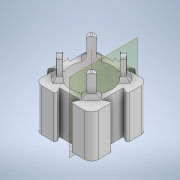
# Autodesk Inventor part: 4x11mmFlatBottom
Saved by Autodesk Inventor 2022.2 (Build 262287010, 287A)
## iProperties
Part Number: 4x11mmFlatBottom
Material: Generic
Document SubType Name: Modeling
Designer: yiunf
Appearance: Default
Author: yiunf
## iProperties of the stored document 4x11mm_3DPrint.ipt
Part Number: 4x11mm_3DPrint
Material: Generic
Document SubType Name: Modeling
Designer: yiunf
Appearance: Default
Author: yiunf
Autodesk Inventor part; units mm, degrees
ref_plane "YZ Plane" through (0, 0, 0) normal (1, 0, 0) x (0, 1, 0)
ref_plane "XZ Plane" through (0, 0, 0) normal (0, 1, 0) x (-1, 0, 0)
ref_plane "XY Plane" through (0, 0, 0) normal (0, 0, 1) x (1, 0, 0)
sketch "Sketch1" plane through (0, 0, 0) normal (0, 1, 0) x (-1, 0, 0)
  line L0 (-20, -20) -> (20, -20)
  line L1 (20, -20) -> (20, 20)
  line L2 (20, 20) -> (-20, 20)
  line L3 (-20, 20) -> (-20, -20)
  line L4 (-20, -20) -> (20, 20) construction
  line L5 (20, -20) -> (-20, 20) construction
  line L6 (20, 0) -> (25, 0)
  line L7 (25, 0) -> (25, 7.5)
  line L8 (20, 0) -> (20, 5)
  line L9 (20, 5) -> (25, 7.5)
  line L10 (25, 0) -> (25, -7.5)
  line L11 (20, 0) -> (20, -5)
  line L12 (20, -5) -> (25, -7.5)
  line L13 (0, -20) -> (5, -20)
  line L14 (0, -20) -> (-5, -20)
  line L15 (0, -20) -> (0, -25)
  line L16 (0, -25) -> (7.5, -25)
  line L17 (7.5, -25) -> (5, -20)
  line L18 (0, -25) -> (-7.5, -25)
  line L19 (-7.5, -25) -> (-5, -20)
  line L20 (-15, 0) -> (-15, -7.5)
  line L21 (-20, -5) -> (-15, -7.5)
  line L22 (-20, 0) -> (-15, 0)
  line L23 (-15, 0) -> (-15, 7.5)
  line L24 (-20, 5) -> (-15, 7.5)
  line L25 (-7.5, 15) -> (-5, 20)
  line L26 (0, 15) -> (-7.5, 15)
  line L27 (0, 20) -> (0, 15)
  line L28 (7.5, 15) -> (5, 20)
  line L29 (0, 15) -> (7.5, 15)
  line L30 (0, -24.75) -> (7.0955, -24.75)
  line L31 (7.0955, -24.75) -> (4.8455, -20.25)
  line L32 (4.8455, -20.25) -> (0, -20.25)
  line L33 (0, -24.75) -> (-7.0955, -24.75)
  line L34 (-7.0955, -24.75) -> (-4.8455, -20.25)
  line L35 (-4.8455, -20.25) -> (0, -20.25)
  line L36 (7.0955, -24.75) -> (4.7205, -20)
  line L37 (-7.0955, -24.75) -> (-4.7205, -20)
  line L38 (24.75, 0) -> (24.75, -7.0955)
  line L39 (24.75, -7.0955) -> (20.25, -4.8455)
  line L40 (20.25, -4.8455) -> (20.25, 0)
  line L41 (24.75, 0) -> (24.75, 7.0955)
  line L42 (24.75, 7.0955) -> (20.25, 4.8455)
  line L43 (20.25, 4.8455) -> (20.25, 0)
  line L44 (24.75, -7.0955) -> (20, -4.7205)
  line L45 (24.75, 7.0955) -> (20, 4.7205)
  line L46 (24.75, 0) -> (23.75, 0)
  line L47 (23.75, 0) -> (23.75, -6.875)
  line L48 (23.75, 0) -> (23.75, 6.875)
  line L49 (0, -24.75) -> (0, -23.75)
  line L50 (0, -23.75) -> (6.875, -23.75)
  line L51 (0, -23.75) -> (-6.875, -23.75)
  point P0 (0, 0)
  point P1 (-4.7205, -20)
  point P2 (20, -4.7205)
  point P3 (20, 4.7205)
  point P4 (23.75, -6.5955)
  point P5 (23.75, 6.5955)
  point P6 (-6.5955, -23.75)
  point P7 (6.5955, -23.75)
  dimension "d0" = 40
  dimension "d1" = 40
  dimension "d2" = 5
  dimension "d3" = 7.5
  dimension "d4" = 5
  dimension "d5" = 7.5
  dimension "d6" = 5
  dimension "d7" = 5
  dimension "d8" = 5
  dimension "d9" = 5
  dimension "d10" = 7.5
  dimension "d11" = 7.5
  dimension "d14" = 40
  dimension "d21" = 40
  dimension "d43" = 0.25
  dimension "d44" = 0.25
  dimension "d45" = 0.25
  dimension "d46" = 0.25
  dimension "d57" = 1
  dimension "d58" = 1
  constraints: 104 end point, 21 point on line, 5 perpendicular, 4 midpoint, 3 horizontal, 3 parallel, 3 vertical, 30 other
  measures "d0" distance of L2.end L1.end
  measures "d1" distance of L1.end L0.end
  measures "d2" distance of L6.start L6.end
  measures "d3" distance of L6.end L7.end
  measures "d4" distance of L6.start L8.end
  measures "d5" distance of L6.end L10.end
  measures "d6" distance of L6.start L11.end
  measures "d7" distance of L13.start L13.end
  measures "d8" distance of L13.start L14.end
  measures "d9" distance of L13.start L15.end
  measures "d10" distance of L15.end L16.end
  measures "d11" distance of L15.end L18.end
  measures "d14" distance of L10.end L20.end
  measures "d21" distance of L18.end L25.start
  measures "d43" distance between parallel lines of L16 L30
  measures "d44" distance between parallel lines of L18 L33
  measures "d45" distance between parallel lines of L10 L38
  measures "d46" distance between parallel lines of L7 L41
  measures "d57" distance of L41.start L46.end
  measures "d58" distance of L33.start L49.end
extrude "Extrusion1" add sketch "Sketch1" along normal blind 30 contours L3 L21 L20 L23 L24 L2 L25 L26 L29 L28 L1 L0 | L0 L15 L35 L37 | L0 L36 L32 L15 | L35 L15 L51 L34 | L32 L31 L50 L15 | L1 L6 L40 L44 | L1 L45 L43 L6 | L40 L6 L47 L39 | L43 L42 L48 L6
sketch "Sketch2" plane through (0, 30, 0) normal (0, 1, 0) x (1, 0, 0)
  line L0 (-20, 20) -> (15, 20)
  line L1 (15, 20) -> (15, -15)
  line L2 (15, -15) -> (-20, -15)
  line L3 (-20, -15) -> (-20, 20)
  circle A0 centre (-2.5, 2.5) radius 14.5
  point P0 (0, 0)
  dimension "d47" = 35
  dimension "d48" = 29
  constraints: 8 end point, 2 parallel, 1 centre point, 1 horizontal, 1 perpendicular
  measures "d47" distance of L0.end L1.end
  measures "d48" diameter of A0
extrude "Extrusion2" cut sketch "Sketch2" against normal blind 25 contours A0
fillet "Fillet1" radius 1 4 edges at (20, 15, -5) (20, 15, 5) (5, 15, 20) (-5, 15, 20)
fillet "Fillet2" radius 5 4 edges at (20, 15, -20) (20, 15, 20) (-20, 15, 20) (-20, 15, -20)
sketch "Sketch3" plane through (0, 30, 0) normal (0, 1, 0) x (1, 0, 0)
  circle A0 centre (-2.5, 2.5) radius 14.5 projected
  circle A1 centre (-2.5, 2.5) radius 14.5
  circle A2 centre (-2.5, 2.5) radius 17.5
  line L0 (-18.4099, 11.3388) -> (6.3388, -13.4099)
  line L1 (6.3388, -13.4099) -> (13.4099, -6.3388)
  line L2 (13.4099, -6.3388) -> (-11.3388, 18.4099)
  line L3 (-11.3388, 18.4099) -> (-18.4099, 11.3388)
  line L4 (-18.4099, 11.3388) -> (13.4099, -6.3388) construction
  line L5 (6.3388, -13.4099) -> (-11.3388, 18.4099) construction
  line L6 (-18.4099, 11.3388) -> (16.5901, 11.3388) construction
  line L7 (8.0912, 16.6267) -> (-16.6267, -8.0912)
  line L8 (-16.6267, -8.0912) -> (-13.0912, -11.6267)
  line L9 (-13.0912, -11.6267) -> (11.6267, 13.0912)
  line L10 (11.6267, 13.0912) -> (8.0912, 16.6267)
  line L11 (8.0912, 16.6267) -> (-13.0912, -11.6267) construction
  line L12 (-16.6267, -8.0912) -> (11.6267, 13.0912) construction
  line L13 (-13.1066, 16.6421) -> (11.6421, -8.1066)
  line L14 (11.6421, -8.1066) -> (8.1066, -11.6421)
  line L15 (8.1066, -11.6421) -> (-16.6421, 13.1066)
  line L16 (-16.6421, 13.1066) -> (-13.1066, 16.6421)
  line L17 (-13.1066, 16.6421) -> (8.1066, -11.6421) construction
  line L18 (11.6421, -8.1066) -> (-16.6421, 13.1066) construction
  point P0 (0, 0)
  point P1 (-2.5, 2.5)
  point P2 (10.4765, 14.2414)
  point P3 (9.2414, 15.4765)
  point P4 (7.9797, 16.5152)
  point P5 (5.8317, 14.3673)
  point P6 (9.3673, 10.8317)
  point P7 (11.5152, 12.9797)
  point P8 (5.8317, -9.3673)
  point P9 (7.9797, -11.5152)
  point P10 (11.5152, -7.9797)
  point P11 (9.3673, -5.8317)
  point P12 (-16.5152, 12.9797)
  point P13 (-14.3673, 10.8317)
  point P14 (-10.8317, 14.3673)
  point P15 (-12.9797, 16.5152)
  point P16 (-12.9797, -11.5152)
  point P17 (-10.8317, -9.3673)
  point P18 (-14.3673, -5.8317)
  point P19 (-16.5152, -7.9797)
  point P20 (-15.4765, -9.2414)
  point P21 (-14.2414, -10.4765)
  dimension "d49" = 35
  dimension "d50" = 45
  dimension "d51" = 10
  dimension "d52" = 5
  dimension "d53" = 5
  constraints: 38 end point, 7 midpoint, 7 parallel, 3 perpendicular, 2 centre point, 2 coincident, 1 equal length, 1 horizontal
  measures "d49" diameter of A2
  measures "d50" angle of L0 L6
  measures "d51" distance of L1.end L0.end
  measures "d52" distance of L8.end L7.end
  measures "d53" distance of L13.end L14.end
extrude "Extrusion3" add sketch "Sketch3" along normal blind 15 contours A0 L7 A2 L10 L9 | L13 A2 L15 A0 | A0 L15 A2 L13 | L9 A2 L8 L7 A0
fillet "Fillet3" radius 2 8 edges at (-11.9057, 45, 10.4412) (-15.4412, 45, 6.9057) (-11.9057, 45, -15.4412) (-15.4412, 45, -11.9057) (6.9057, 45, 10.4412) (10.4412, 45, 6.9057) (10.4412, 45, -11.9057) (6.9057, 45, -15.4412)
sketch "Sketch4" plane through (0, 30, 0) normal (0, 1, 0) x (1, 0, 0)
  point P0 (0, 0)
ref_plane "Work Plane1" through (6.5955, 0, -23.75) normal (-1, 0, 0) x (0, 1, 0)
sketch "Sketch5" plane through (6.5955, 0, -23.75) normal (-1, 0, 0) x (0, 1, 0)
  line L0 (0, -3.75) -> (30, -3.75) projected
  line L1 (15, -3.75) -> (15, 2)
  line L2 (0, 0) -> (30, 0) projected
  arc A0 (30, 0) -> (0, 0) centre (15, -55.25) ccw
  line L3 (15, 2) -> (15, 1)
  line L4 (30, 0) -> (25, 0)
  line L5 (25, 0) -> (5, 0)
  arc A1 (25, 0) -> (5, 0) centre (15, -49.5) ccw
  point P0 (0, -23.75)
  dimension "d60" = 5.75
  dimension "d61" = 1
  dimension "d62" = 5
  dimension "d63" = 20
  constraints: 8 end point, 6 point on circle, 3 point on line, 2 centre point, 1 midpoint, 1 vertical
  measures "d60" distance of L1.start L1.end
  measures "d61" distance of L1.end L3.end
  measures "d62" distance of L2.end L4.end
  measures "d63" distance of L4.end L5.end
extrude "Extrusion4" add sketch "Sketch5" along normal blind 13.191 contours A1 L2 A0 L1 | L1 A0 L2 A1
fillet "Fillet4" radius 2 2 edges at (0, 30, -23.75) (0, 0, -23.75)
pattern_circular "Circular Pattern1" count 2 over 90 about axis through (0, 30, 0) along (0, 1, 0) of "Extrusion4", "Fillet4"
chamfer "Chamfer1" distance 2.5 angle 45 16 edges at (-15.4412, 30, 6.9057) (-16.0106, 30, 8.6227) (-14.8589, 30, 9.8589) (-13.6227, 30, 11.0106) (-11.9057, 30, 10.4412) (6.9057, 30, 10.4412) (9.8744, 30, 9.8744) (10.4412, 30, 6.9057) (6.9057, 30, -15.4412) (8.6227, 30, -16.0106) (9.8589, 30, -14.8589) (11.0106, 30, -13.6227) (10.4412, 30, -11.9057) (-11.9057, 30, -15.4412) (-14.8744, 30, -14.8744) (-15.4412, 30, -11.9057)
body "Solid1"
